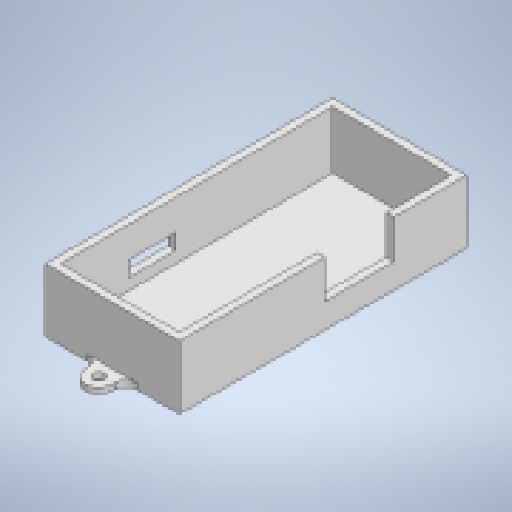
# Autodesk Inventor part: Caja
Saved by Autodesk Inventor 2024 (Build 280153000, 153)
## iProperties
Created: 2025-05-11
Part Number: Caja
Material: Genérico
Document SubType Name: Modeling
Designer: sergi
Density: 1 g/cm^3
Appearance: Valor por defecto
Author: sergi
Autodesk Inventor part; units mm, degrees
ref_plane "YZ Plane" through (0, 0, 0) normal (1, 0, 0) x (0, 1, 0)
ref_plane "XZ Plane" through (0, 0, 0) normal (0, 1, 0) x (-1, 0, 0)
ref_plane "XY Plane" through (0, 0, 0) normal (0, 0, 1) x (1, 0, 0)
sketch "Boceto1" plane through (0, 0, 0) normal (0, 1, 0) x (-1, 0, 0)
  line L0 (-15.2057, -35) -> (14.7943, -35)
  line L1 (14.7943, -35) -> (14.7943, 35)
  line L2 (14.7943, 35) -> (-15.2057, 35)
  line L3 (-15.2057, 35) -> (-15.2057, -35)
  line L4 (-15.2057, -35) -> (14.7943, 35) construction
  line L5 (14.7943, -35) -> (-15.2057, 35) construction
  line L6 (15.2943, 35.5) -> (15.2943, -35.5)
  line L7 (15.2943, -35.5) -> (-15.7057, -35.5)
  line L8 (-15.7057, -35.5) -> (-15.7057, 35.5)
  line L9 (-15.7057, 35.5) -> (15.2943, 35.5)
  line L10 (17.2943, -37.5) -> (17.2943, 37.5)
  line L11 (17.2943, 37.5) -> (-17.7057, 37.5)
  line L12 (-17.7057, 37.5) -> (-17.7057, -37.5)
  line L13 (-17.7057, -37.5) -> (17.2943, -37.5)
  point P0 (0, 0)
  point P1 (-0.2057, 0)
  dimension "d0" = 30
  dimension "d1" = 70
  dimension "d2" = 0.5
  dimension "d3" = 2
  constraints: 28 end point, 6 parallel, 3 perpendicular, 2 midpoint, 1 horizontal, 6 other
  measures "d0" distance of L2.end L1.end
  measures "d1" distance of L1.end L0.end
  measures "d2" distance between parallel lines of L1 L6
  measures "d3" distance between parallel lines of L6 L10
extrude "Extrusión1" add sketch "Boceto1" along normal blind 15 contours L13 L12 L11 L10
sketch "Boceto2" plane through (0, 0, 0) normal (0, -1, 0) x (1, 0, 0)
  line L0 (-17.2943, 37.5) -> (17.7057, 37.5) projected
  line L1 (-17.2943, -37.5) -> (-17.2943, 37.5) projected
  line L2 (17.7057, -37.5) -> (-17.2943, -37.5) projected
  line L3 (17.7057, 37.5) -> (17.7057, -37.5) projected
  line L4 (-15.2943, 35.5) -> (-15.2943, -35.5) projected
  line L5 (15.7057, 35.5) -> (-15.2943, 35.5) projected
  line L6 (15.7057, -35.5) -> (15.7057, 35.5) projected
  line L7 (-15.2943, -35.5) -> (15.7057, -35.5) projected
  point P0 (0, 0)
extrude "Extrusión2" add sketch "Boceto2" along normal blind 1.5 contours L0 L3 L2 L1 | L5 L6 L7 L4
sketch "Boceto3" plane through (0, -1.5, 0) normal (0, -1, 0) x (1, 0, 0)
  line L0 (-17.2943, -37.5) -> (17.7057, -37.5) projected
  line L1 (17.7057, -37.5) -> (17.7057, 37.5) projected
  line L2 (17.7057, 37.5) -> (-17.2943, 37.5) projected
  line L3 (-17.2943, 37.5) -> (-17.2943, -37.5) projected
  line L4 (-17.2943, 37.5) -> (17.7057, 37.5)
  line L5 (17.7057, 37.5) -> (17.7057, 44.5)
  line L6 (17.7057, 44.5) -> (-17.2943, 44.5)
  line L7 (-17.2943, 44.5) -> (-17.2943, 37.5)
  circle A0 centre (0.2057, 41) radius 1.5
  arc A1 (3.6377, 40.3136) -> (-3.2839, 40.7308) centre (0.2057, 41) ccw
  arc A2 (-3.5482, 41.7508) -> (-3.2839, 40.7308) centre (-6.2751, 40.5) ccw
  arc A3 (3.6953, 40.7308) -> (6.6864, 37.5) centre (6.6864, 40.5) ccw
  line L8 (3.6377, 40.3136) -> (17.7057, 37.5)
  line L9 (-17.2943, 44.5) -> (-3.2263, 41.6864)
  line L10 (-1.2652, 41.2942) -> (1.6766, 40.7058)
  point P0 (0, 0)
  point P1 (3.6929, 40.3026)
  point P2 (-6.2751, 37.5)
  dimension "d8" = 7
  dimension "d9" = 35
  dimension "d10" = 3
  dimension "d11" = 6
  dimension "d12" = 6
  dimension "d13" = 7
  constraints: 14 end point, 10 point on circle, 4 centre point, 4 tangent, 2 parallel, 2 point on line, 1 coincident, 1 horizontal, 1 midpoint, 1 perpendicular
  measures "d8" distance of L5.end L4.end
  measures "d9" distance of L5.end L6.end
  measures "d10" diameter of A0
  measures "d11" diameter of A2
  measures "d12" diameter of A3
  measures "d13" diameter of A1
extrude "Extrusión3" add sketch "Boceto3" against normal blind 1.5 contours A2 A1 L8 A3 L2
mirror "Simetría1" about plane through (0, 0, 0) normal (0, 0, 1) of "Extrusión3"
sketch "Boceto4" plane through (-15.2943, 15, 35.5) normal (1, 0, 0) x (0, 0, -1)
  line L0 (0, -15) -> (71, -15) projected
  line L1 (71, -15) -> (71, 0) projected
  line L2 (0, 0) -> (71, 0) projected
  line L3 (0, -15) -> (0, 0) projected
  line L4 (0, -15) -> (30, -15)
  line L5 (30, -15) -> (30, -12)
  line L6 (30, -12) -> (18, -12)
  line L7 (18, -12) -> (30, -12)
  line L8 (30, -12) -> (30, -8)
  line L9 (30, -8) -> (18, -8)
  line L10 (18, -8) -> (18, -12)
  point P0 (35.5, -15)
  dimension "d16" = 30
  dimension "d17" = 3
  dimension "d18" = 12
  constraints: 14 end point, 2 horizontal, 2 parallel, 2 perpendicular, 1 point on line
  measures "d16" distance of L0.start L4.end
  measures "d17" distance of L4.end L5.end
  measures "d18" distance of L5.end L6.end
extrude "Extrusión4" cut sketch "Boceto4" against normal up to surface (2 mm away) contours L6 L10 L9 L8
sketch "Boceto5" plane through (15.7057, 15, -35.5) normal (-1, 0, 0) x (0, 0, 1)
  line L0 (71, -15) -> (71, 0) projected
  line L1 (71, 0) -> (17, 0)
  line L2 (0, 0) -> (71, 0) projected
  line L3 (71, -15) -> (17, -15)
  line L4 (0, -15) -> (71, -15) projected
  line L5 (17, -15) -> (17, -10)
  line L6 (17, -10) -> (17, 0)
  line L7 (17, -10) -> (35, -10)
  line L8 (35, -10) -> (35, 0)
  line L9 (35, 0) -> (17, 0)
  line L10 (17, 0) -> (17, -10)
  point P0 (35.5, -15)
  point P1 (17, 0)
  dimension "d21" = 54
  dimension "d22" = 54
  dimension "d23" = 5
  dimension "d24" = 10
  dimension "d25" = 18
  dimension "d26" = 10
  constraints: 16 end point, 3 point on line, 2 parallel, 2 perpendicular, 1 horizontal
  measures "d21" distance of L0.end L1.end
  measures "d22" distance of L0.start L3.end
  measures "d23" distance of L3.end L5.end
  measures "d24" distance of L5.end L6.end
  measures "d25" distance of L9.end L8.end
  measures "d26" distance of L8.end L7.end
extrude "Extrusión5" cut sketch "Boceto5" against normal blind 10 contours L8 L7 L6 L1
